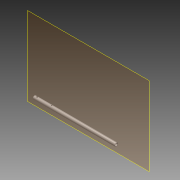
# Autodesk Inventor part: 12 inch pipe
Saved by Autodesk Inventor 2014 SP1 (Build 180222100, 222)
## iProperties
Created: 2014-01-12
Part Number: 12 inch pipe
Material: Aluminum
Document SubType Name: Modeling
Designer: Michael
Mass: 116.606 g
Surface Area: 543.196 cm^2
Volume: 43.0282 cm^3
Density: 2.71 g/cm^3
Appearance: Satin
Author: Michael
Autodesk Inventor part; units mm, degrees
ref_plane "YZ Plane" through (0, 0, 0) normal (1, 0, 0) x (0, 1, 0)
sketch "Sketch1" plane through (0, 0, 0) normal (0, 0, 1) x (1, 0, 0)
  line L0 (0, 0) -> (304.8, 0)
  arc A0 (304.8, 0) -> (406.4, 101.6) centre (304.8, 101.6) ccw
  line L1 (406.4, 101.6) -> (406.4, 152.4)
  line L2 (304.8, 0) -> (304.8, 101.6) construction
  line L3 (304.8, 101.6) -> (406.4, 101.6) construction
  arc A1 (406.4, 152.4) -> (304.8, 254) centre (304.8, 152.4) ccw
  line L4 (406.4, 152.4) -> (304.8, 152.4) construction
  line L5 (304.8, 152.4) -> (304.8, 254) construction
  line L6 (304.8, 254) -> (203.2, 254)
  circle A2 centre (668.9835, 281.347) radius 317.5 construction
  dimension "d0" = 304.8
  dimension "d1" = 101.6
  dimension "d2" = 50.8
  dimension "d3" = 101.6
  dimension "d4" = 101.6
  dimension "d7" = 635
  constraints: 14 end point, 4 perpendicular, 4 point on circle, 3 centre point, 2 parallel, 2 tangent, 1 horizontal
  measures "d0" distance of L0.start L0.end
  measures "d1" radius of A0
  measures "d2" distance of L1.start L1.end
  measures "d3" radius of A1
  measures "d4" distance of L5.end L6.end
  measures "d7" diameter of A2
sketch "Sketch2" plane through (0, 0, 0) normal (1, 0, 0) x (0, 1, 0)
  circle A0 centre (0, 0) radius 6.35
  circle A1 centre (0, 0) radius 4.7625
  dimension "d5" = 12.7
  dimension "d8" = 9.525
  constraints: 2 centre point, 2 coincident
  measures "d5" diameter of A0
  measures "d8" diameter of A1
sweep "Sweep1" add profiles "Sketch2" path "Sketch1"
ref_plane "Work Plane1" through (0, 6.35, 0) normal (0, 1, 0) x (-1, 0, 0)
sketch "Sketch3" plane through (0, 6.35, 0) normal (0, 1, 0) x (-1, 0, 0)
  circle A0 centre (-63.5, 0) radius 2.0828
  line L0 (0, 6.35) -> (-304.8, 6.35) projected
  line L1 (0, -6.35) -> (-304.8, -6.35) projected
  line L2 (0, -6.35) -> (0, 6.35) projected
  circle A1 centre (-9.525, 0) radius 2.4638
  point P0 (0, 0)
  dimension "d9" = 4.1656
  dimension "d10" = 63.5
  dimension "d11" = 6.35
  dimension "d14" = 4.9276
  dimension "d15" = 9.525
  dimension "d16" = 6.35
  constraints: 2 centre point
  measures "d9" diameter of A0
  measures "d10" distance from line of A0.centre L2
  measures "d11" distance from line of L1 A0.centre
  measures "d14" diameter of A1
  measures "d15" distance from line of L2 A1.centre
  measures "d16" distance from line of L1 A1.centre
extrude "Extrusion1" cut sketch "Sketch3" against normal blind 25.4
ref_plane "Work Plane2" through (0, 0, 6.35) normal (0, 0, 1) x (1, 0, 0)
sketch "Sketch4" plane through (0, 0, 6.35) normal (0, 0, 1) x (1, 0, 0)
  line L0 (0, 0) -> (304.8, 0)
  line L1 (304.8, 0) -> (304.8, 213.1624)
  line L2 (304.8, 213.1624) -> (152.4, 213.1624)
  line L3 (152.4, 213.1624) -> (152.4, 273.9577)
  line L4 (152.4, 273.9577) -> (436.2539, 273.9577)
  line L5 (436.2539, 273.9577) -> (436.2539, -18.5171)
  line L6 (436.2539, -18.5171) -> (304.8, -18.5171)
  line L7 (304.8, -18.5171) -> (304.8, 15.9884)
  dimension "d17" = 304.8
  constraints: 16 end point, 5 parallel, 1 horizontal, 1 perpendicular, 1 point on line
  measures "d17" distance of L0.start L0.end
extrude "Extrusion2" cut sketch "Sketch4" against normal blind 25.4
body "Solid1"
